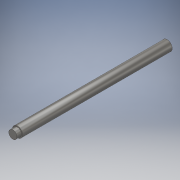
# Autodesk Inventor part: Motor Axle
Saved by Autodesk Inventor 2019.4 (Build 234330000, 330)
## iProperties
Created: 2019-10-19
Part Number: Motor Axle
Material: Stainless Steel
Document SubType Name: Modeling
Designer: admin
Density: 8 g/cm^3
Appearance: Semi-Polished
Author: admin
Autodesk Inventor part; units mm, degrees
ref_plane "YZ Plane" through (0, 0, 0) normal (1, 0, 0) x (0, 1, 0)
ref_plane "XZ Plane" through (0, 0, 0) normal (0, 1, 0) x (-1, 0, 0)
ref_plane "XY Plane" through (0, 0, 0) normal (0, 0, 1) x (1, 0, 0)
sketch "Sketch1" plane through (0, 0, 0) normal (1, 0, 0) x (0, 1, 0)
  line L0 (0, 0) -> (4, 0)
  line L1 (4, 0) -> (4, -4.5)
  line L2 (4, -4.5) -> (5, -4.5)
  line L3 (5, -4.5) -> (5, -150.3)
  line L4 (5, -150.3) -> (0, -150.3)
  line L5 (0, -150.3) -> (0, 0)
  dimension "d0" = 5
  dimension "d1" = 4
  dimension "d2" = 4.5
  dimension "d3" = 150.3
  constraints: 12 end point, 4 perpendicular, 2 horizontal
  measures "d0" distance between parallel lines of L3 L5
  measures "d1" distance between parallel lines of L5 L1
  measures "d2" distance of L0.end L1.end
  measures "d3" distance of L4.end L0.start
revolve "Revolution1" add sketch "Sketch1" angle 360 about axis through (0, 0, -150.3) along (0, 0, 1)
sketch "Sketch2" plane through (0, 0, -150.3) normal (0, 0, -1) x (-1, 0, 0)
  line L0 (0, 4) -> (3.4641, 2)
  line L1 (3.4641, 2) -> (3.4641, -2)
  line L2 (3.4641, -2) -> (0, -4)
  line L3 (0, -4) -> (-3.4641, -2)
  line L4 (-3.4641, -2) -> (-3.4641, 2)
  line L5 (-3.4641, 2) -> (0, 4)
  point P0 (0, 0)
  point P1 (0, 0)
  dimension "d5" = 8
  constraints: 12 end point, 1 coincident, 13 other
  measures "d5" distance of L2.end L0.start
extrude "Extrusion1" [suppressed]
body "Solid1"
